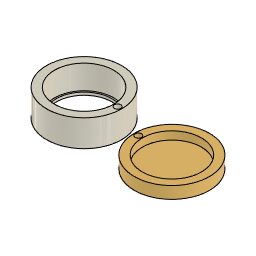
YankeeTreatHolder (Autodesk Fusion 360 design; units mm, degrees)
Autodesk Fusion 360 part; units mm, degrees
sketch "Sketch1" plane through (0, 0, 0) normal (0, 0, 1) x (1, 0, 0)
  circle A0 centre (51.5404, 40.9839) radius 35
  circle A1 centre (51.5404, 40.9839) radius 40
  line L0 (51.5404, 40.9839, 0) -> (51.5404, 40.9839, 3.5)
  circle A2 through (88.5404, 40.9839, 3.5) (33.0404, 73.0268, 3.5) (33.0404, 8.941, 3.5)
  circle A3 through (91.5404, 40.9839, 3.5) (31.5404, 75.6249, 3.5) (31.5404, 6.3429, 3.5)
  dimension "d1" = 70
  dimension "d2" = 80
  dimension "d3" = 3.5
  dimension "d4" = 74
  dimension "d5" = 80
  constraint concentric A0 A1
  constraint coincident A0.centre A1.centre
  measures "d1" diameter of A0
  measures "d2" diameter of A1
  measures "d3" distance of A0.centre A1.centre
extrude "Extrude1" add sketch "Sketch1" along normal blind 3.5 makes body 1
extrude "Extrude2" add sketch "Sketch1" along normal blind 30 contours A3 in plane through (0, 0, 3.5) normal (0, 0, 1) bodies 1
move_face "OffsetFaces1" offset 2 1 faces at (11.5901, 42.9777, 11.1667) on bodies 1
move_face "OffsetFaces2" offset 5 1 faces at (9.7491, 36.8021, 11.1667) on bodies 1
sketch "Sketch2" plane through (0, 0, 33.5) normal (0, 0, 1) x (-1, 0, 0)
  circle A0 centre (-51.5404, -40.9839) radius 37
  circle A1 centre (-51.5404, -40.9839) radius 47
  circle A2 centre (-93.5404, -40.9839) radius 4.05
  dimension "d12" = 8.1
  measures "d12" diameter of A2
extrude "Extrude3" cut sketch "Sketch2" against normal blind 10 contours A2 bodies 1
extrude "Extrude4" add 1 faces at (92.1955, 50.5833, 33.5) along direction (0, 0, 1) blind 10 separate body on bodies 1 makes body 2
sketch "Sketch3" plane through (0, 0, 43.5) normal (0, 0, 1) x (-1, 0, 0)
  circle A0 centre (-93.5404, -40.9839) radius 4.05
  circle A1 centre (-51.5404, -40.9839) radius 37
  circle A2 centre (-51.5404, -40.9839) radius 47
  circle A3 centre (-51.5404, -40.9839) radius 47
  constraint concentric A1 A3
extrude "Extrude5" add sketch "Sketch3" along normal blind 5 contours A0 | A1 | A2 A3 bodies 2
move_body "Move1" bodies 2 to x (1, 0, 0) y (0, 1, 0) z (0, 0, 1) at (110, 0, -33.5)
move_body "Move2" bodies 2 to x (-1, 0, 0) y (0, 1, 0) z (0, 0, -1) at (323.0807, 0, 15)
